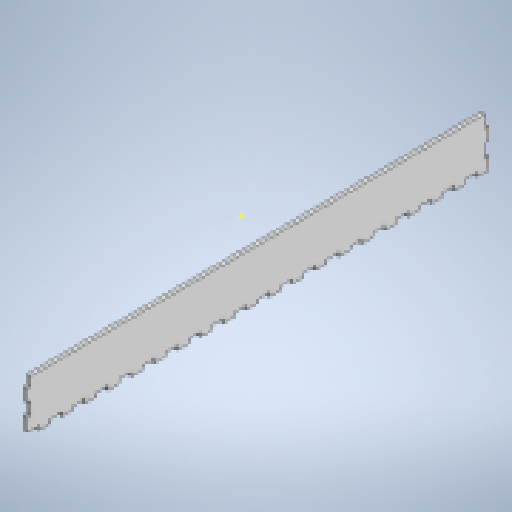
# Autodesk Inventor part: LeftBaseWall
Saved by Autodesk Inventor 2024 (Build 280153000, 153)
## iProperties
Created: 2023-09-08
Part Number: LeftBaseWall
Material: Generic
Document SubType Name: Modeling
Designer: Bruno
Density: 1 g/cm^3
Appearance: Default
Author: Bruno
Autodesk Inventor part; units mm, degrees
ref_plane "YZ Plane" through (0, 0, 0) normal (1, 0, 0) x (0, 1, 0)
ref_plane "XZ Plane" through (0, 0, 0) normal (0, 1, 0) x (-1, 0, 0)
ref_plane "XY Plane" through (0, 0, 0) normal (0, 0, 1) x (1, 0, 0)
sketch "Sketch2" plane through (0, 0, 0) normal (1, 0, 0) x (0, 1, 0)
  line L0 (-30.375, -191.625) -> (-30.375, -188.625)
  line L1 (-30.375, -188.625) -> (-39.5, -188.625)
  line L2 (-39.5, -188.625) -> (-39.5, -191.625)
  line L3 (-39.5, -191.625) -> (-48.625, -191.625)
  line L4 (-30.375, -191.625) -> (-21.25, -191.625)
  line L5 (-21.25, -191.625) -> (-21.25, -188.625)
  line L6 (-21.25, -188.625) -> (-12.125, -188.625)
  line L7 (-48.625, -191.625) -> (-48.625, -182.5)
  line L8 (-48.625, -182.5) -> (-45.625, -182.5)
  line L9 (-45.625, -182.5) -> (-45.625, -173.375)
  line L10 (-45.625, -173.375) -> (-48.625, -173.375)
  line L11 (-48.625, -173.375) -> (-48.625, -164.25)
  line L12 (-48.625, -164.25) -> (-45.625, -164.25)
  line L13 (-45.625, -164.25) -> (-45.625, -155.125)
  line L14 (-45.625, -155.125) -> (-48.625, -155.125)
  line L15 (-48.625, -155.125) -> (-48.625, -146)
  line L16 (-48.625, -146) -> (-45.625, -146)
  line L17 (-45.625, -146) -> (-45.625, -136.875)
  line L18 (-45.625, -136.875) -> (-48.625, -136.875)
  line L19 (-48.625, -136.875) -> (-48.625, -127.75)
  line L20 (-48.625, -127.75) -> (-45.625, -127.75)
  line L21 (-45.625, -127.75) -> (-45.625, -118.625)
  line L22 (-45.625, -118.625) -> (-48.625, -118.625)
  line L23 (-48.625, -118.625) -> (-48.625, -109.5)
  line L24 (-48.625, -109.5) -> (-45.625, -109.5)
  line L25 (-45.625, -109.5) -> (-45.625, -100.375)
  line L26 (-45.625, -100.375) -> (-48.625, -100.375)
  line L27 (-48.625, -100.375) -> (-48.625, -91.25)
  line L28 (-48.625, -91.25) -> (-45.625, -91.25)
  line L29 (-45.625, -91.25) -> (-45.625, -82.125)
  line L30 (-45.625, -82.125) -> (-48.625, -82.125)
  line L31 (-48.625, -82.125) -> (-48.625, -73)
  line L32 (-48.625, -73) -> (-45.625, -73)
  line L33 (-45.625, -73) -> (-45.625, -63.875)
  line L34 (-45.625, -63.875) -> (-48.625, -63.875)
  line L35 (-48.625, -63.875) -> (-48.625, -54.75)
  line L36 (-48.625, -54.75) -> (-45.625, -54.75)
  line L37 (-45.625, -54.75) -> (-45.625, -45.625)
  line L38 (-45.625, -45.625) -> (-48.625, -45.625)
  line L39 (-48.625, -45.625) -> (-48.625, -36.5)
  line L40 (-48.625, -36.5) -> (-45.625, -36.5)
  line L41 (-45.625, -36.5) -> (-45.625, -27.375)
  line L42 (-45.625, -27.375) -> (-48.625, -27.375)
  line L43 (-48.625, -27.375) -> (-48.625, -18.25)
  line L44 (-48.625, -18.25) -> (-45.625, -18.25)
  line L45 (-45.625, -18.25) -> (-45.625, -9.125)
  line L46 (-45.625, -9.125) -> (-48.625, -9.125)
  line L47 (-48.625, -9.125) -> (-48.625, 0)
  line L48 (-48.625, 0) -> (-45.625, 0)
  line L49 (-45.625, 0) -> (-45.625, 9.125)
  line L50 (-45.625, 9.125) -> (-48.625, 9.125)
  line L51 (-48.625, 9.125) -> (-48.625, 18.25)
  line L52 (-48.625, 18.25) -> (-45.625, 18.25)
  line L53 (-45.625, 18.25) -> (-45.625, 27.375)
  line L54 (-45.625, 27.375) -> (-48.625, 27.375)
  line L55 (-48.625, 27.375) -> (-48.625, 36.5)
  line L56 (-48.625, 36.5) -> (-45.625, 36.5)
  line L57 (-45.625, 36.5) -> (-45.625, 45.625)
  line L58 (-45.625, 45.625) -> (-48.625, 45.625)
  line L59 (-48.625, 45.625) -> (-48.625, 54.75)
  line L60 (-48.625, 54.75) -> (-45.625, 54.75)
  line L61 (-45.625, 54.75) -> (-45.625, 63.875)
  line L62 (-45.625, 63.875) -> (-48.625, 63.875)
  line L63 (-48.625, 63.875) -> (-48.625, 73)
  line L64 (-48.625, 73) -> (-45.625, 73)
  line L65 (-45.625, 73) -> (-45.625, 82.125)
  line L66 (-45.625, 82.125) -> (-48.625, 82.125)
  line L67 (-48.625, 82.125) -> (-48.625, 91.25)
  line L68 (-48.625, 91.25) -> (-45.625, 91.25)
  line L69 (-45.625, 91.25) -> (-45.625, 100.375)
  line L70 (-45.625, 100.375) -> (-48.625, 100.375)
  line L71 (-48.625, 100.375) -> (-48.625, 109.5)
  line L72 (-48.625, 109.5) -> (-45.625, 109.5)
  line L73 (-45.625, 109.5) -> (-45.625, 118.625)
  line L74 (-45.625, 118.625) -> (-48.625, 118.625)
  line L75 (-48.625, 118.625) -> (-48.625, 127.75)
  line L76 (-48.625, 127.75) -> (-45.625, 127.75)
  line L77 (-45.625, 127.75) -> (-45.625, 136.875)
  line L78 (-45.625, 136.875) -> (-48.625, 136.875)
  line L79 (-48.625, 136.875) -> (-48.625, 146)
  line L80 (-48.625, 146) -> (-45.625, 146)
  line L81 (-45.625, 146) -> (-45.625, 155.125)
  line L82 (-45.625, 155.125) -> (-48.625, 155.125)
  line L83 (-48.625, 155.125) -> (-48.625, 164.25)
  line L84 (-48.625, 164.25) -> (-45.625, 164.25)
  line L85 (-45.625, 164.25) -> (-45.625, 173.375)
  line L86 (-12.125, -188.625) -> (-12.125, -191.625)
  line L87 (-12.125, -191.625) -> (-3, -191.625)
  line L88 (-3, -191.625) -> (-3, -182.5)
  line L89 (-3, -182.5) -> (0, -182.5)
  line L90 (0, -182.5) -> (0, -173.375)
  line L91 (0, -173.375) -> (-3, -173.375)
  line L92 (-3, -173.375) -> (-3, -164.25)
  line L93 (-3, -164.25) -> (0, -164.25)
  line L94 (0, -164.25) -> (0, -155.125)
  line L95 (0, -155.125) -> (-3, -155.125)
  line L96 (-3, -155.125) -> (-3, -146)
  line L97 (-3, -146) -> (0, -146)
  line L98 (0, -146) -> (0, -136.875)
  line L99 (0, -136.875) -> (-3, -136.875)
  line L100 (-3, -136.875) -> (-3, -127.75)
  line L101 (-3, -127.75) -> (0, -127.75)
  line L102 (0, -127.75) -> (0, -118.625)
  line L103 (0, -118.625) -> (-3, -118.625)
  line L104 (-3, -118.625) -> (-3, -109.5)
  line L105 (-3, -109.5) -> (0, -109.5)
  line L106 (0, -109.5) -> (0, -100.375)
  line L107 (0, -100.375) -> (-3, -100.375)
  line L108 (-3, -100.375) -> (-3, -91.25)
  line L109 (-3, -91.25) -> (0, -91.25)
  line L110 (0, -91.25) -> (0, -82.125)
  line L111 (0, -82.125) -> (-3, -82.125)
  line L112 (-3, -82.125) -> (-3, -73)
  line L113 (-3, -73) -> (0, -73)
  line L114 (0, -73) -> (0, -63.875)
  line L115 (0, -63.875) -> (-3, -63.875)
  line L116 (-3, -63.875) -> (-3, -54.75)
  line L117 (-3, -54.75) -> (0, -54.75)
  line L118 (0, -54.75) -> (0, -45.625)
  line L119 (0, -45.625) -> (-3, -45.625)
  line L120 (-3, -45.625) -> (-3, -36.5)
  line L121 (-3, -36.5) -> (0, -36.5)
  line L122 (0, -36.5) -> (0, -27.375)
  line L123 (0, -27.375) -> (-3, -27.375)
  line L124 (-3, -27.375) -> (-3, -18.25)
  line L125 (-3, -18.25) -> (0, -18.25)
  line L126 (0, -18.25) -> (0, -9.125)
  line L127 (0, -9.125) -> (-3, -9.125)
  line L128 (-3, -9.125) -> (-3, 0)
  line L129 (-3, 0) -> (0, 0)
  line L130 (0, 0) -> (0, 9.125)
  line L131 (0, 9.125) -> (-3, 9.125)
  line L132 (-3, 9.125) -> (-3, 18.25)
  line L133 (-3, 18.25) -> (0, 18.25)
  line L134 (0, 18.25) -> (0, 27.375)
  line L135 (0, 27.375) -> (-3, 27.375)
  line L136 (-3, 27.375) -> (-3, 36.5)
  line L137 (-3, 36.5) -> (0, 36.5)
  line L138 (0, 36.5) -> (0, 45.625)
  line L139 (0, 45.625) -> (-3, 45.625)
  line L140 (-3, 45.625) -> (-3, 54.75)
  line L141 (-3, 54.75) -> (0, 54.75)
  line L142 (0, 54.75) -> (0, 63.875)
  line L143 (0, 63.875) -> (-3, 63.875)
  line L144 (-3, 63.875) -> (-3, 73)
  line L145 (-3, 73) -> (0, 73)
  line L146 (0, 73) -> (0, 82.125)
  line L147 (0, 82.125) -> (-3, 82.125)
  line L148 (-3, 82.125) -> (-3, 91.25)
  line L149 (-3, 91.25) -> (0, 91.25)
  line L150 (0, 91.25) -> (0, 100.375)
  line L151 (0, 100.375) -> (-3, 100.375)
  line L152 (-3, 100.375) -> (-3, 109.5)
  line L153 (-3, 109.5) -> (0, 109.5)
  line L154 (0, 109.5) -> (0, 118.625)
  line L155 (0, 118.625) -> (-3, 118.625)
  line L156 (-3, 118.625) -> (-3, 127.75)
  line L157 (-3, 127.75) -> (0, 127.75)
  line L158 (0, 127.75) -> (0, 136.875)
  line L159 (0, 136.875) -> (-3, 136.875)
  line L160 (-3, 136.875) -> (-3, 146)
  line L161 (-3, 146) -> (0, 146)
  line L162 (0, 146) -> (0, 155.125)
  line L163 (0, 155.125) -> (-3, 155.125)
  line L164 (-3, 155.125) -> (-3, 164.25)
  line L165 (-3, 164.25) -> (0, 164.25)
  line L166 (0, 164.25) -> (0, 173.375)
  line L167 (-18.25, 173.375) -> (-18.25, 170.375)
  line L168 (-18.25, 170.375) -> (-9.125, 170.375)
  line L169 (-9.125, 170.375) -> (-9.125, 173.375)
  line L170 (-9.125, 173.375) -> (0, 173.375)
  line L171 (-18.25, 173.375) -> (-27.375, 173.375)
  line L172 (-27.375, 173.375) -> (-27.375, 170.375)
  line L173 (-27.375, 170.375) -> (-36.5, 170.375)
  line L174 (-36.5, 170.375) -> (-36.5, 173.375)
  line L175 (-36.5, 173.375) -> (-45.625, 173.375)
  point P0 (-3, -173.375)
  point P1 (-3, -155.125)
  point P2 (-3, -136.875)
  point P3 (-3, -118.625)
  point P4 (-3, -100.375)
  point P5 (-3, -82.125)
  point P6 (-3, -63.875)
  point P7 (-3, -45.625)
  point P8 (-3, -27.375)
  point P9 (-3, -9.125)
  point P10 (-3, 9.125)
  point P11 (-3, 27.375)
  point P12 (-3, 45.625)
  point P13 (-3, 63.875)
  point P14 (-3, 82.125)
  point P15 (-3, 100.375)
  point P16 (-3, 118.625)
  point P17 (-3, 136.875)
  point P18 (0, 173.375)
  dimension "d1" = 3
  dimension "d4" = 3
  dimension "d6" = 18.25
  dimension "d9" = 18.25
  dimension "d15" = 9.125
  dimension "d22" = 3
  dimension "d23" = 18.25
  dimension "d24" = 18.25
  dimension "d26" = 3
  dimension "d27" = 9.125
  constraints: 352 end point, 38 point on line, 23 perpendicular, 22 equal length, 9 vertical, 6 coincident, 2 collinear, 2 horizontal, 322 other
  measures "d1" distance of L1.end L2.end
  measures "d4" distance of L7.end L8.end
  measures "d6" distance of L10.end L3.end
  measures "d9" distance of L7.end L11.end
  measures "d15" distance of L2.end L3.end
  measures "d22" distance of L89.start L90.start
  measures "d23" distance of L91.end L88.start
  measures "d24" distance of L89.start L92.end
  measures "d26" distance of L169.start L169.end
  measures "d27" distance of L169.end L170.end
extrude "Extrusion1" add sketch "Sketch2" along normal blind 3
body "Solid1"
